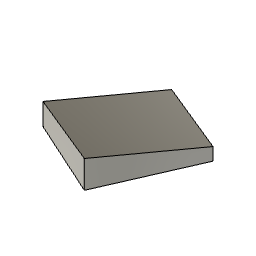
motor_place (Autodesk Fusion 360 design; units mm, degrees)
Autodesk Fusion 360 part; units mm, degrees
sketch "Sketch1" plane through (0, 0, 0) normal (1, 0, 0) x (0, 1, 0)
  line L0 (0, 0) -> (0, 60)
  line L1 (0, 0) -> (270, 0)
  line L2 (270, 0) -> (270, 15)
  line L3 (0, 60) -> (270, 15)
  dimension "d1" = 60
  dimension "d2" = 270
  dimension "d3" = 15
  constraint coincident L0.start L1.start
  constraint vertical L0
  constraint perpendicular L0 L1
  constraint perpendicular L1 L2
  measures "d1" distance of L0.start L0.end
  measures "d2" distance of L0.start L1.end
  measures "d3" distance of L1.end L2.end
extrude "Extrude1" add sketch "Sketch1" along normal blind 250
sketch "Sketch2" plane through (0, 0, 0) normal (0, 0, -1) x (1, 0, 0)
  line L0 (0, 0) -> (0, -270)
  line L1 (0, -270) -> (250, -270)
  line L2 (250, -270) -> (250, 0)
  line L3 (250, 0) -> (0, 0)
  line L4 (250, -270) -> (250, -195)
  line L5 (250, 0) -> (165, 0)
  line L6 (0, 0) -> (0, -75)
  line L7 (250, -195) -> (165, 0)
  line L8 (165, 0) -> (0, -75)
  line L9 (0, -270) -> (85, -270)
  line L10 (0, -75) -> (85, -270)
  line L11 (85, -270) -> (250, -195)
  line L12 (0, -270) -> (250, -270)
  line L13 (250, -270) -> (250, 0)
  line L14 (250, 0) -> (0, 0)
  line L15 (0, 0) -> (0, -270)
  dimension "d6" = 75
  dimension "d7" = 85
  dimension "d8" = 75
  dimension "d9" = 85
  constraint coincident L1.end L2.start
  constraint perpendicular L1 L4
  constraint coincident L2.end L3.start
  constraint perpendicular L2 L5
  constraint coincident L0.start L3.end
  constraint perpendicular L3 L6
  constraint coincident L0.end L1.start
  constraint perpendicular L0 L9
  constraint horizontal L12
  constraint vertical L13
  constraint horizontal L14
  constraint vertical L15
  measures "d6" distance of L1.end L4.end
  measures "d7" distance of L2.end L5.end
  measures "d8" distance of L0.start L6.end
  measures "d9" distance of L0.end L9.end
extrude "Extrude2" cut sketch "Sketch2" against normal blind 100 contours L0 L3 L6 L8 L14 L15 | L0 L1 L9 L10 L12 L15 | L2 L3 L5 L7 L13 L14 | L1 L2 L4 L11 L12 L13
